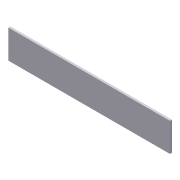
# Autodesk Inventor part: FE-00018-03
Saved by Autodesk Inventor 2012 (Build 160160000, 160)
## iProperties
Company: FIRST
Created: 2008-05-30
Part Number: FE-00018-03
Document SubType Name: Modeling
Designer: dfoster
Density: 1 g/cm^3
Description: Mounting Plate
Mass: 283.189 g
Surface Area: 966.934 cm^2
Volume: 283.189 cm^3
Material: Default
Title: Mounting Plate
Author: dfoster
Autodesk Inventor part; units mm, degrees
ref_plane "YZ Plane" through (0, 0, 0) normal (1, 0, 0) x (0, 1, 0)
ref_plane "XZ Plane" through (0, 0, 0) normal (0, 1, 0) x (-1, 0, 0)
ref_plane "XY Plane" through (0, 0, 0) normal (0, 0, 1) x (1, 0, 0)
sketch "Sketch1" plane through (0, 0, 0) normal (0, 0, 1) x (1, 0, 0)
  line L0 (-25.4, 90.4875) -> (476.25, 90.4875)
  line L1 (476.25, 90.4875) -> (476.25, 1.5875)
  line L2 (476.25, 1.5875) -> (-25.4, 1.5875)
  line L3 (-25.4, 1.5875) -> (-25.4, 90.4875)
  dimension "d0" = 88.9
  dimension "d1" = 501.65
  constraints: 8 end point, 2 parallel, 1 horizontal, 1 perpendicular
  measures "d0" distance of L2.end L0.start
  measures "d1" distance of L1.end L2.end
extrude "Extrusion1" add sketch "Sketch1" along normal blind 6.35
body "Solid1"
